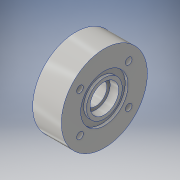
# Autodesk Inventor part: 0.375 in hole
Saved by Autodesk Inventor 2016 (Build 200138000, 138)
## iProperties
Created: 2016-06-27
Part Number: 0.375 in hole
Material: Aluminum 6061
Document SubType Name: Modeling
Designer: Jonathan
Density: 2.7 g/cm^3
Appearance: Aluminum - Flat
Author: Jonathan
Autodesk Inventor part; units mm, degrees
ref_plane "YZ Plane" through (0, 0, 0) normal (1, 0, 0) x (0, 1, 0)
sketch "Sketch1" plane through (0, 0, 0) normal (1, 0, 0) x (0, 1, 0)
  circle A0 centre (0, 0) radius 19.05
  dimension "d0" = 38.1
  constraints: 1 centre point, 1 coincident
  measures "d0" diameter of A0
extrude "Extrusion1" add sketch "Sketch1" along normal blind 12.7
sketch "Sketch10" plane through (12.7, 0, 0) normal (1, 0, 0) x (0, 0, -1)
  point P0 (0, 0)
  point P1 (0, 0)
  constraints: 1 coincident
hole "Hole4" at (12.7, 0, 0) direction (-1, 0, 0) diameter 12.7 depth 3.81
ref_plane "Work Plane2" through (8.89, 0, 0) normal (1, 0, 0) x (0, 0, -1)
hole "Hole1" at (8.89, 0, 0) direction (-1, 0, 0) diameter 9.9219 depth 4.7625
ref_plane "Work Plane1" through (-12.7, 0, 0) normal (1, 0, 0) x (0, 0, -1)
sketch "Sketch5" plane through (0, 0, 0) normal (1, 0, 0) x (0, 1, 0)
  line L0 (0, 9) -> (0, -9)
  circle A0 centre (0, 0) radius 19.05 projected
  line L1 (-10.795, 0) -> (10.795, 0)
  line L2 (-10.795, 8.89) -> (-10.795, -8.89)
  dimension "d37" = 18
  dimension "d45" = 21.59
  dimension "d46" = 17.78
  constraints: 6 end point, 4 coincident, 3 midpoint, 2 vertical, 1 parallel, 1 perpendicular
  measures "d37" distance of L0.start L0.end
  measures "d45" distance of L1.start L1.end
  measures "d46" distance of L2.start L2.end
hole "Hole2" at (0, 0, -9) direction (1, 0, 0) diameter 2.159 depth 8.8646 tip angle 118
sketch "Sketch6" plane through (0, 0, 0) normal (-1, 0, 0) x (0, 0, 1)
  circle A0 centre (0, 0) radius 0.5715
  dimension "d34" = 1.143
  constraints: 1 centre point, 1 coincident
  measures "d34" diameter of A0
hole "Hole5" at (0, 0, 0) direction (1, 0, 0) diameter 1 end through all
mirror "Mirror1" about plane through (0, 0, 0) normal (0, 0, 1) of "Hole2"
hole "Hole3" at (0, -10.795, 8.89) at (0, -10.795, -8.89) direction (1, 0, 0) diameter 2.9464 end through all clearance for "Flat Head Machine Screw (82)" size "#4" standard "Ansi Unified Screw Threads"
mirror "Mirror2" about plane through (0, 0, 0) normal (0, 1, 0) of "Hole3"
sketch "Sketch9" plane through (0, 0, 0) normal (0, 1, 0) x (-1, 0, 0)
  line L0 (-11.4554, -7.9375) -> (-12.7, -7.9375)
  line L1 (-12.7, -7.9375) -> (-12.7, -10.4775)
  line L2 (-12.7, -10.4775) -> (-11.4554, -10.4775)
  line L3 (-11.4554, -10.4775) -> (-11.4554, -7.9375)
  line L4 (2.54, 0) -> (-15.24, 0) projected
  line L5 (-12.7, 19.05) -> (-12.7, -19.05) projected
  point P0 (0, 0)
  dimension "d55" = 2.54
  dimension "d56" = 1.2446
  dimension "d59" = 7.9375
  constraints: 8 end point, 2 parallel, 1 collinear, 1 perpendicular
  measures "d55" distance of L2.end L0.start
  measures "d56" distance of L1.end L2.end
  measures "d59" distance between parallel lines of L4 L0
revolve "Revolution1" cut sketch "Sketch9" angle 360 about axis through (-10, 0, 0) along (1, 0, 0)
body "Solid1"
